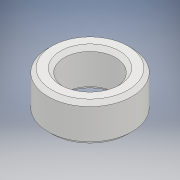
# Autodesk Inventor part: Entretoise
Saved by Autodesk Inventor 2017 (Build 210142000, 142)
## iProperties
Company: FABLAB Frenchmakers
Part Number: Entretoise
Project: 1420 VAUBAN 3D XL
Material: Plastique ABS
Catalog Web Link: http://www.frenchmakers.com/
Document SubType Name: Modeling
Designer: FABLAB Frenchmakers
Mass: 0.29924 g
Surface Area: 3.64648 cm^2
Volume: 0.282302 cm^3
Density: 1.06 g/cm^3
Appearance: Lisse - Blanc
Stock Number: 1420-03-01
Autodesk Inventor part; units mm, degrees
ref_plane "YZ Plane" through (0, 0, 0) normal (1, 0, 0) x (0, 1, 0)
ref_plane "XZ Plane" through (0, 0, 0) normal (0, 1, 0) x (-1, 0, 0)
ref_plane "XY Plane" through (0, 0, 0) normal (0, 0, 1) x (1, 0, 0)
sketch "Esquisse1" plane through (0, 0, 0) normal (0, 0, 1) x (1, 0, 0)
  circle A0 centre (0, 0) radius 3.375
  circle A1 centre (0, 0) radius 5.5
  dimension "d0" = 6.75
  dimension "d1" = 11
  constraints: 2 centre point, 2 coincident
  measures "d0" diameter of A0
  measures "d1" diameter of A1
extrude "Extrusion1" add sketch "Esquisse1" along normal blind 5
chamfer "Chanfrein1" distance 0.5 angle 45 4 edges at (-5.5, 0, 0) (-3.375, 0, 0) (-5.5, 0, 5) (-3.375, 0, 5)
